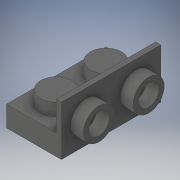
# Autodesk Inventor part: Two Sided Piece
Saved by Autodesk Inventor 2017 (Build 210142000, 142)
## iProperties
Created: 2018-05-17
Part Number: Two Sided Piece
Material: ABS Plastic
Document SubType Name: Modeling
Designer: Kyle
Density: 1.06 g/cm^3
Appearance: Gray
Author: Kyle
Autodesk Inventor part; units mm, degrees
ref_plane "YZ Plane" through (0, 0, 0) normal (1, 0, 0) x (0, 1, 0)
ref_plane "XZ Plane" through (0, 0, 0) normal (0, 1, 0) x (-1, 0, 0)
ref_plane "XY Plane" through (0, 0, 0) normal (0, 0, 1) x (1, 0, 0)
sketch "Sketch1" plane through (0, 0, 0) normal (0, 1, 0) x (-1, 0, 0)
  line L0 (0, 0) -> (7.7978, 0)
  line L1 (7.7978, 0) -> (7.7978, -15.5956)
  line L2 (7.7978, -15.5956) -> (0, -15.5956)
  line L3 (0, -15.5956) -> (0, 0)
  dimension "d0" = 7.7978
  dimension "d8" = 15.5956
  constraints: 8 end point, 2 parallel, 1 horizontal, 1 perpendicular
  measures "d0" distance of L1.end L2.end
  measures "d8" distance of L0.end L1.end
extrude "Extrusion1" add sketch "Sketch1" along normal blind 3.236
sketch "Sketch2" plane through (0, 3.236, 0) normal (0, 1, 0) x (1, 0, 0)
  line L0 (0, 0) -> (0, 15.5956) construction
  line L1 (0, 0) -> (-3.8989, 0) construction
  line L2 (-3.8989, 0) -> (-3.8989, 3.8989) construction
  line L3 (-3.8989, 3.8989) -> (0, 3.8989) construction
  line L4 (0, 3.8989) -> (0, 0) construction
  circle A0 centre (-3.8989, 3.8989) radius 2.4498
  dimension "d11" = 3.8989
  dimension "d12" = 3.8989
  dimension "d13" = 4.8997
  constraints: 8 end point, 2 parallel, 1 centre point, 1 coincident, 1 horizontal, 1 perpendicular
  measures "d11" distance of L2.end L3.end
  measures "d12" distance of L1.end L2.end
  measures "d13" diameter of A0
extrude "Extrusion2" add sketch "Sketch2" along normal blind 1.9837
pattern_linear "Rectangular Pattern1" count 2 spacing 7.7978 along (0, 0, -1) of "Extrusion2"
shell "Shell1" thickness 1.4732 removed faces 1 at (-2.5993, 0, -5.1985)
sketch "Sketch3" plane through (-6.3246, 1.7628, -1.4732) normal (0, -1, 0) x (1, 0, 0)
  circle A0 centre (2.4257, -2.4257) radius 2.4498 construction
  circle A1 centre (2.4257, -10.2235) radius 2.4498 construction
  circle A2 centre (2.4257, -2.4257) radius 0.9766 construction
  line L0 (2.4257, -2.4257) -> (2.4257, -10.2235) construction
  circle A3 centre (2.4257, -6.3246) radius 1.4491
  circle A4 centre (2.4257, -6.3246) radius 0.6198
  point P0 (6.3246, 1.4732)
  dimension "d20" = 1.2395
  constraints: 2 centre point, 2 end point, 1 coincident, 1 midpoint, 1 vertical
  measures "d20" diameter of A4
extrude "Extrusion3" add sketch "Sketch3" along normal up to surface (1.7628 mm away)
sketch "Sketch4" plane through (0, 0, 0) normal (1, 0, 0) x (0, 0, -1)
  line L0 (0, 0) -> (15.5956, 0)
  line L1 (15.5956, 0) -> (15.5956, 7.7978)
  line L2 (15.5956, 7.7978) -> (0, 7.7978)
  line L3 (0, 7.7978) -> (0, 0)
  dimension "d23" = 15.5956
  dimension "d24" = 7.7978
  constraints: 8 end point, 2 parallel, 1 horizontal, 1 perpendicular
  measures "d23" distance of L2.end L1.end
  measures "d24" distance of L1.end L0.end
extrude "Extrusion4" add sketch "Sketch4" along normal blind 0.809
sketch "Sketch5" plane through (0.809, 0, 0) normal (1, 0, 0) x (0, 0, -1)
  line L0 (0, 0) -> (15.5956, 0) construction
  line L1 (0, 0) -> (3.8989, 0) construction
  line L2 (3.8989, 0) -> (3.8989, 3.8989) construction
  line L3 (3.8989, 3.8989) -> (0, 3.8989) construction
  line L4 (0, 3.8989) -> (0, 0) construction
  circle A0 centre (3.8989, 3.8989) radius 2.4498
  dimension "d27" = 3.8989
  dimension "d28" = 3.8989
  dimension "d29" = 4.8997
  constraints: 8 end point, 2 parallel, 1 centre point, 1 coincident, 1 horizontal, 1 perpendicular
  measures "d27" distance of L3.end L2.end
  measures "d28" distance of L2.end L1.end
  measures "d29" diameter of A0
extrude "Extrusion5" add sketch "Sketch5" along normal blind 1.9837
sketch "Sketch6" plane through (2.7927, 3.8989, -3.8989) normal (1, 0, 0) x (0, 0, -1)
  circle A0 centre (0, 0) radius 2.4498 construction
  circle A1 centre (0, 0) radius 1.618
  point P0 (-3.8989, -3.8989)
  dimension "d32" = 3.236
  constraints: 1 centre point, 1 coincident
  measures "d32" diameter of A1
extrude "Extrusion6" cut sketch "Sketch6" against normal blind 1.9837
pattern_linear "Rectangular Pattern2" count 2 spacing 7.7978 along (0, 0, -1) of "Extrusion6", "Extrusion5"
equation "\"d0\" = d1"
equation "\"d8\" = 2 * d1"
equation "\"d9\" = d2"
equation "\"d11\" = 0.5 * d1"
equation "\"d12\" = 0.5 * d1"
equation "\"d13\" = d4"
equation "\"d14\" = d5"
equation "\"d18\" = d1"
equation "\"d19\" = d6"
equation "\"d20\" = d7"
equation "\"d21\" = d5"
equation "\"d23\" = 2 * d1"
equation "\"d24\" = d1"
equation "\"d25\" = 0.25 * d2"
equation "\"d27\" = 0.5 * d1"
equation "\"d28\" = 0.5 * d1"
equation "\"d29\" = d4"
equation "\"d30\" = d5"
equation "\"d32\" = d2"
equation "\"d33\" = d5"
equation "\"d37\" = d1"
equation "\"d1\" = 7.7978"
equation "\"d2\" = 3.23596"
equation "\"d3\" = 9.60882"
equation "\"d4\" = 4.89966"
equation "\"d5\" = 1.98374"
equation "\"d6\" = 1.4732"
equation "\"d7\" = 1.23952"
body "Solid1"
